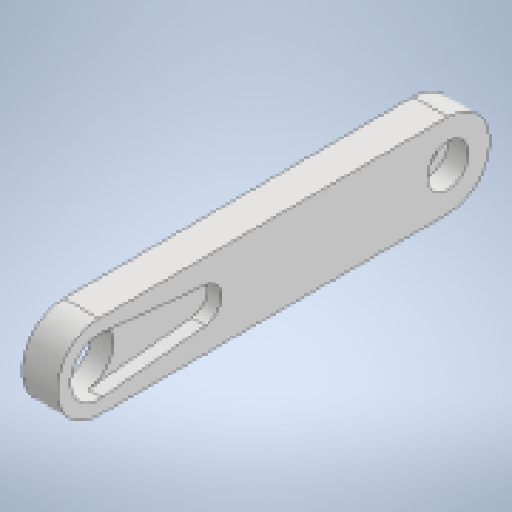
# Autodesk Inventor part: belka
Saved by Autodesk Inventor 2023 (Build 270158000, 158)
## iProperties
Created: 2024-05-12
Part Number: belka
Material: Ogólny
Document SubType Name: Modeling
Designer: kamil
Density: 1 g/cm^3
Appearance: Domyślna
Author: kamil
Autodesk Inventor part; units mm, degrees
ref_plane "YZ Plane" through (0, 0, 0) normal (1, 0, 0) x (0, 1, 0)
ref_plane "XZ Plane" through (0, 0, 0) normal (0, 1, 0) x (-1, 0, 0)
ref_plane "XY Plane" through (0, 0, 0) normal (0, 0, 1) x (1, 0, 0)
sketch "Szkic1" plane through (0, 0, 0) normal (1, 0, 0) x (0, 1, 0)
  line L0 (9.9771, 19.755) -> (9.9771, -30.245) construction
  line L1 (3.9771, 19.755) -> (3.9771, -30.245)
  line L2 (15.9771, -30.245) -> (15.9771, 19.755)
  arc A0 (15.9771, 19.755) -> (3.9771, 19.755) centre (9.9771, 19.755) ccw
  arc A1 (3.9771, -30.245) -> (15.9771, -30.245) centre (9.9771, -30.245) ccw
  circle A2 centre (9.9771, 19.755) radius 1.6
  circle A3 centre (9.9771, -30.245) radius 1.6
  point P0 (0, 0)
  point P1 (9.9771, -5.245)
  dimension "d0" = 50
  dimension "d1" = 12
  dimension "d2" = 3.2
  dimension "d3" = 3.2
  constraints: 8 end point, 4 centre point, 4 point on circle, 4 tangent, 2 coincident, 1 midpoint, 1 parallel, 1 vertical
  measures "d0" distance of L0.start L0.end
  measures "d1" diameter of A1
  measures "d2" diameter of A2
  measures "d3" diameter of A3
extrude "Wyciągnięcie proste1" add sketch "Szkic1" along normal blind 3
sketch "Szkic4" plane through (3, 0, 0) normal (1, 0, 0) x (0, 0, -1)
  circle A0 centre (-19.755, 9.9771) radius 1.6 projected
  arc A1 (-19.38, 13.7083) -> (-19.38, 6.2459) centre (-19.755, 9.9771) ccw
  arc A2 (-4.53, 7.7383) -> (-4.53, 12.2158) centre (-4.755, 9.9771) ccw
  line L0 (-19.38, 13.7083) -> (-4.53, 12.2158)
  line L1 (-19.38, 6.2459) -> (-4.53, 7.7383)
  line L2 (-4.5, 12.5143) -> (-19.35, 14.0068)
  arc A3 (-19.35, 14.0068) -> (-19.35, 5.9474) centre (-19.755, 9.9771) ccw
  line L3 (-19.35, 5.9474) -> (-4.5, 7.4398)
  arc A4 (-4.5, 7.4398) -> (-4.5, 12.5143) centre (-4.755, 9.9771) ccw
  circle A5 centre (-19.755, 9.9771) radius 4.05
  arc A6 (30.245, 3.9771) -> (30.245, 15.9771) centre (30.245, 9.9771) ccw projected
  line L4 (30.245, 15.9771) -> (-19.755, 15.9771) projected
  arc A7 (-19.755, 15.9771) -> (-19.755, 3.9771) centre (-19.755, 9.9771) ccw projected
  line L5 (-19.755, 3.9771) -> (30.245, 3.9771) projected
  circle A8 centre (30.245, 9.9771) radius 1.6 projected
  circle A9 centre (-19.755, 9.9771) radius 1.6 projected
  point P0 (0, 0)
  point P1 (-19.35, 14.0068)
  dimension "d12" = 7.5
  dimension "d13" = 4.5
  dimension "d14" = 15
  dimension "d15" = 0.3
  constraints: 8 end point, 8 point on circle, 5 centre point, 4 tangent, 2 coincident, 1 concentric, 1 horizontal alignment, 3 other
  measures "d12" diameter of A1
  measures "d13" diameter of A2
  measures "d14" distance of A2.centre A0.centre
  measures "d15" distance between parallel lines of L0 L2
extrude "Wyciągnięcie proste4" add sketch "Szkic4" along normal blind 2 contours L5 A7 L4 A6
extrude "Wyciągnięcie proste5" cut sketch "Szkic4" against normal blind 3 contours A0 | L0 A5 L1 A1 | A1 L1 A5 A3 L0
sketch "Szkic5" plane through (5, 0, 0) normal (1, 0, 0) x (0, 0, -1)
  circle A0 centre (30.245, 9.9771) radius 1.6 projected
  circle A1 centre (30.245, 9.9771) radius 3
  point P0 (0, 0)
  dimension "d20" = 6
  constraints: 1 centre point, 1 coincident
  measures "d20" diameter of A1
extrude "Wyciągnięcie proste6" cut sketch "Szkic5" against normal blind 3 contours A0 | A1
